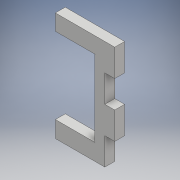
# Autodesk Inventor part: muñeca7
Saved by Autodesk Inventor 2018 (Build 220112000, 112)
## iProperties
Created: 2020-03-11
Part Number: muñeca7
Material: Genérico
Document SubType Name: Modeling
Designer: david
Density: 1 g/cm^3
Appearance: Valor por defecto
Author: david
Autodesk Inventor part; units mm, degrees
ref_plane "YZ Plane" through (0, 0, 0) normal (1, 0, 0) x (0, 1, 0)
ref_plane "XZ Plane" through (0, 0, 0) normal (0, 1, 0) x (-1, 0, 0)
ref_plane "XY Plane" through (0, 0, 0) normal (0, 0, 1) x (1, 0, 0)
sketch "Boceto1" plane through (0, 0, 0) normal (0, 1, 0) x (-1, 0, 0)
  line L0 (0, 0) -> (0, -8.25)
  line L1 (0, -8.25) -> (3, -8.25)
  line L2 (3, -8.25) -> (3, -16.5)
  line L3 (3, -16.5) -> (0, -16.5)
  line L4 (0, -16.5) -> (0, -24.75)
  line L5 (0, -24.75) -> (3, -24.75)
  line L6 (3, -24.75) -> (3, -33)
  line L7 (3, -33) -> (20, -33)
  line L8 (20, 0) -> (0, 0)
  line L9 (20, -28) -> (8, -28)
  line L10 (8, -28) -> (8, -5)
  line L11 (8, -5) -> (20, -5)
  line L12 (20, -33) -> (20, -28)
  line L13 (20, -5) -> (20, 0)
  dimension "d0" = 8.25
  dimension "d1" = 3
  dimension "d3" = 8.25
  constraints: 28 end point, 8 perpendicular, 4 point on line, 3 vertical, 2 horizontal
  measures "d0" distance of L0.start L0.end
  measures "d1" distance of L0.end L1.end
  measures "d3" distance of L3.end L4.end
extrude "Extrusión1" add sketch "Boceto1" along normal blind 3
sketch "Boceto2" plane through (0, 0, 0) normal (0, -1, 0) x (1, 0, 0)
  line L0 (-8, -28) -> (-8, -5) projected
  line L1 (-8, -5) -> (-8, -28)
  line L2 (-8, -28) -> (-6, -28)
  line L3 (-6, -28) -> (-6, -5)
  line L4 (-6, -5) -> (-8, -5)
  line L5 (-20, 0) -> (-20, -5)
  line L6 (-20, -5) -> (-18, -5)
  line L7 (-18, -5) -> (-18, 0)
  line L8 (-18, 0) -> (-20, 0)
  line L9 (-20, -33) -> (-20, -28)
  line L10 (-20, -28) -> (-18, -28)
  line L11 (-18, -28) -> (-18, -33)
  line L12 (-18, -33) -> (-20, -33)
  constraints: 24 end point, 6 perpendicular, 3 vertical, 1 point on line
extrude "Extrusión2" cut sketch "Boceto2" against normal blind 10
sketch "Boceto5" plane through (0, 0, 0) normal (0, -1, 0) x (1, 0, 0)
  line L0 (-18, -5) -> (-6, -5) projected
  line L1 (-18, -5) -> (-18, -4.832)
  line L2 (-18, -5) -> (-18, 0) projected
  line L3 (-18, -4.832) -> (-6, -4.832)
  line L4 (-6, -5) -> (-6, -28) projected
  line L5 (-6, -4.832) -> (-6, -5)
  line L6 (-6, -5) -> (-18, -5)
  point P0 (0, 0)
  dimension "d22" = 0.168
  constraints: 8 end point, 3 perpendicular, 1 point on line
  measures "d22" distance of L0.start L1.end
extrude "Extrusión4" cut sketch "Boceto5" against normal blind 3
